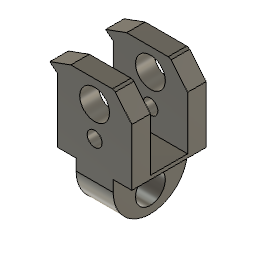
ankle (Autodesk Fusion 360 design; units mm, degrees)
part number: 2025-10-29-11-47-36-964
Autodesk Fusion 360 part; units mm, degrees
sketch "Sketch1" plane through (0, 0, 0) normal (1, 0, 0) x (0, 1, 0)
  line L0 (0, 0) -> (-25.4, 0)
  line L1 (-25.4, 0) -> (-25.4, 43.18)
  line L2 (-25.4, 43.18) -> (-19.05, 43.18)
  line L3 (0, 0) -> (0, 43.18)
  line L4 (0, 43.18) -> (-6.35, 43.18)
  line L5 (-6.35, 43.18) -> (-6.35, 17.78)
  line L6 (-19.05, 43.18) -> (-19.05, 17.7768)
  line L7 (-19.05, 17.7768) -> (-6.35, 17.78)
  circle A0 centre (-12.7, 7.62) radius 5.08
  dimension "d1" = 25.4
  dimension "d2" = 43.18
  dimension "d3" = 6.35
  dimension "d5" = 25.4
  dimension "d6" = 10.16
  dimension "d7" = 12.7
  dimension "d8" = 7.62
  dimension "d10" = 6.35
  dimension "d11" = 12.7
  dimension "d12" = 43.18
  constraint coincident L0.start L3.start
  constraint horizontal L0
  constraint perpendicular L0 L1
  constraint perpendicular L1 L2
  constraint perpendicular L0 L3
  constraint perpendicular L3 L4
  constraint perpendicular L4 L5
  constraint perpendicular L2 L6
  measures "d1" distance of L0.start L0.end
  measures "d2" distance of L0.end L1.end
  measures "d3" distance of L1.end L2.end
  measures "d5" distance of L4.end L5.end
  measures "d6" diameter of A0
  measures "d7" distance of L3 A0.centre
  measures "d8" distance of L0 A0.centre
  measures "d10" distance of L3.end L4.end
  measures "d11" distance of L5.end L6.end
  measures "d12" distance of L0 L4
extrude "Extrude1" add sketch "Sketch1" along normal blind 25.4
sketch "Sketch2" plane through (25.4, 0, 0) normal (1, 0, 0) x (0, 1, 0)
  circle A0 centre (-12.7, 7.62) radius 5.08
  line L0 (0, 0) -> (0, 43.18)
  line L1 (0, 43.18) -> (-6.35, 43.18)
  line L2 (-6.35, 43.18) -> (-6.35, 17.78)
  line L3 (-6.35, 17.78) -> (-19.05, 17.7768)
  line L4 (-19.05, 17.7768) -> (-19.05, 43.18)
  line L5 (-19.05, 43.18) -> (-25.4, 43.18)
  line L6 (-25.4, 43.18) -> (-25.4, 0)
  line L7 (-25.4, 0) -> (0, 0)
  line L8 (-25.4, 0) -> (0, 0)
  line L9 (0, 0) -> (0, 16.51)
  line L10 (0, 16.51) -> (-25.4, 16.51)
  line L11 (-25.4, 16.51) -> (-25.4, 0)
  dimension "d28" = 16.51
  constraint horizontal L8
  constraint vertical L9
  constraint horizontal L10
  constraint vertical L11
  constraint coincident L0 L9.end
  constraint coincident L6.end L7.start
  measures "d28" distance of L0.start L9.end
extrude "Extrude2" cut sketch "Sketch2" against normal blind 6.3551 contours L0 L6 L7 L8 L9 L10 L11
sketch "Sketch3" plane through (0, 0, 0) normal (-1, 0, 0) x (0, -1, 0)
  circle A0 centre (12.7, 7.62) radius 5.08
  line L0 (0, 43.18) -> (0, 0)
  line L1 (0, 0) -> (25.4, 0)
  line L2 (25.4, 0) -> (25.4, 43.18)
  line L3 (25.4, 43.18) -> (19.05, 43.18)
  line L4 (19.05, 43.18) -> (19.05, 17.7768)
  line L5 (19.05, 17.7768) -> (6.35, 17.78)
  line L6 (6.35, 17.78) -> (6.35, 43.18)
  line L7 (6.35, 43.18) -> (0, 43.18)
  line L8 (0, 0) -> (25.4, 0)
  line L9 (25.4, 0) -> (25.4, 16.51)
  line L10 (25.4, 16.51) -> (0, 16.51)
  line L11 (0, 16.51) -> (0, 0)
  dimension "d29" = 16.51
  constraint horizontal L8
  constraint vertical L9
  constraint horizontal L10
  constraint vertical L11
  constraint coincident L2 L9.end
  constraint coincident L0.end L1.start
  measures "d29" distance of L8 L10
extrude "Extrude3" cut sketch "Sketch3" against normal blind 6.3551 contours L0 L1 L2 L8 L9 L10 L11
sketch "Sketch4" plane through (0, -25.4, 0) normal (0, -1, 0) x (1, 0, 0)
  line L0 (6.3551, 16.51) -> (6.3551, 0)
  line L1 (6.3551, 0) -> (19.0449, 0)
  line L2 (19.0449, 0) -> (19.0449, 16.51)
  line L3 (19.0449, 16.51) -> (25.4, 16.51)
  line L4 (25.4, 16.51) -> (25.4, 43.18)
  line L5 (25.4, 43.18) -> (0, 43.18)
  line L6 (0, 43.18) -> (0, 16.51)
  line L7 (0, 16.51) -> (6.3551, 16.51)
  line L8 (0, 43.18) -> (25.4422, 43.18)
  line L9 (25.4422, 43.18) -> (25.4422, 17.78)
  line L10 (25.4422, 17.78) -> (0, 17.78)
  line L11 (0, 17.78) -> (0, 43.18)
  circle A0 centre (12.7, 25.4) radius 2.54
  circle A1 centre (12.7, 35.56) radius 5.08
  dimension "d19" = 25.4
  dimension "d20" = 5.08
  dimension "d22" = 12.7
  dimension "d23" = 10.16
  dimension "d24" = 7.62
  dimension "d25" = 12.7
  dimension "d47" = 10.16
  constraint horizontal L8
  constraint vertical L9
  constraint horizontal L10
  constraint vertical L11
  constraint coincident L5.end L6.start
  measures "d19" distance of L5.end L10.end
  measures "d20" diameter of A0
  measures "d22" distance of L11 A0.centre
  measures "d23" diameter of A1
  measures "d24" distance of L8 A1.centre
  measures "d25" distance of L11 A1.centre
  measures "d47" distance of A0.centre A1.centre
extrude "Extrude4" cut sketch "Sketch4" against normal blind 40.64 contours A0 | A1
fillet "Fillet1" radius 12.7 2 edges at (12.7, -25.4, 0) (12.7, 0, 0)
chamfer "Chamfer1" distance 6.0452 angle 50 2 edges at (25.4, -22.225, 43.18) (25.4, -3.175, 43.18) measured on face at (8.4667, -23.2833, 43.18) measured on face at (8.4667, -2.1167, 43.18)
chamfer "Chamfer2" distance 4.572 angle 20 1 edges at (0, -3.175, 43.18) measured on face at (12.9032, -2.1167, 43.18)
chamfer "Chamfer3" distance 4.572 angle 20 1 edges at (0, -22.225, 43.18) measured on face at (12.9032, -23.2833, 43.18)
sketch "Sketch5" plane through (0, -25.4, 0) normal (0, -1, 0) x (1, 0, 0)
  line L0 (4.572, 43.18) -> (0, 41.5159)
  line L1 (0, 41.5159) -> (0, 16.51)
  line L2 (0, 16.51) -> (6.3551, 16.51)
  line L3 (6.3551, 16.51) -> (6.3551, 12.7)
  line L4 (6.3551, 12.7) -> (19.0449, 12.7)
  line L5 (19.0449, 12.7) -> (19.0449, 16.51)
  line L6 (19.0449, 16.51) -> (25.4, 16.51)
  line L7 (25.4, 16.51) -> (25.4, 35.9756)
  line L8 (25.4, 35.9756) -> (19.3548, 43.18)
  line L9 (19.3548, 43.18) -> (4.572, 43.18)
  circle A0 centre (12.7, 35.56) radius 5.08
  circle A1 centre (12.7, 25.4) radius 2.54
  line L10 (0, 41.5159) -> (-2.6255, 40.5603)
  line L11 (-2.6255, 40.5603) -> (0, 38.3573)
  dimension "d38" = 2.794
  dimension "d39" = 60
  constraint coincident L0.end L1.start
  constraint parallel L0 L10
  constraint coincident L1 L11.end
  measures "d38" distance of L0.end L10.end
  measures "d39" angle of L10 L11
extrude "Extrude5" add sketch "Sketch5" against normal blind 6.35 contours L1 L10 L11
sketch "Sketch6" plane through (0, 0, 0) normal (0, 1, 0) x (-1, 0, 0)
  line L0 (0, 41.5159) -> (-4.572, 43.18)
  line L1 (-4.572, 43.18) -> (-19.3548, 43.18)
  line L2 (-19.3548, 43.18) -> (-25.4, 35.9756)
  line L3 (-25.4, 35.9756) -> (-25.4, 16.51)
  line L4 (-25.4, 16.51) -> (-19.0449, 16.51)
  line L5 (-19.0449, 16.51) -> (-19.0449, 12.7)
  line L6 (-19.0449, 12.7) -> (-6.3551, 12.7)
  line L7 (-6.3551, 12.7) -> (-6.3551, 16.51)
  line L8 (-6.3551, 16.51) -> (0, 16.51)
  line L9 (0, 16.51) -> (0, 41.5159)
  circle A0 centre (-12.7, 25.4) radius 2.54
  circle A1 centre (-12.7, 35.56) radius 5.08
  line L10 (0, 41.5159) -> (2.6255, 40.5603)
  line L11 (2.6255, 40.5603) -> (0, 38.354)
  line L12 (0, 38.354) -> (0, 41.5159)
  dimension "d42" = 2.794
  constraint coincident L0.start L9.end
  constraint parallel L0 L10
  constraint coincident L9 L11.end
  measures "d42" distance of L0.start L10.end
extrude "Extrude6" add sketch "Sketch6" against normal blind 6.35 contours L9 L10 L11 L12
fillet "Fillet2" radius 1.27 2 edges at (19.3548, -22.225, 43.18) (19.3548, -3.175, 43.18)
